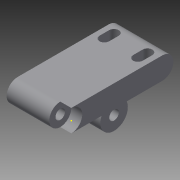
# Autodesk Inventor part: armv2
Saved by Autodesk Inventor 2015 (Build 190159000, 159)
## iProperties
Created: 2015-02-01
Part Number: armv2
Material: Generic
Document SubType Name: Modeling
Designer: Jumziey
Density: 1 g/cm^3
Appearance: Default
Author: Jumziey
Autodesk Inventor part; units mm, degrees
ref_plane "XZ Plane" through (0, 0, 0) normal (0, 1, 0) x (-1, 0, 0)
ref_plane "XY Plane" through (0, 0, 0) normal (0, 0, 1) x (1, 0, 0)
sketch "Sketch1" plane through (0, 0, 0) normal (1, 0, 0) x (0, 1, 0)
  circle A0 centre (0, 0) radius 1.75
  arc A1 (0, 4) -> (0, -4) centre (0, 0) ccw
  line L0 (0, 0) -> (15.55, 0) construction
  line L1 (15.55, -4) -> (15.55, -6) construction
  line L2 (15.55, 0) -> (33.1, 0) construction
  arc A2 (33.1, -4) -> (33.1, 4) centre (33.1, 0) ccw
  line L3 (0, 4) -> (33.1, 4)
  arc A3 (10.9674, -4) -> (20.1326, -4) centre (15.55, -6) ccw
  circle A4 centre (15.55, -6) radius 1.75
  line L4 (0, -4) -> (10.9674, -4)
  line L5 (20.1326, -4) -> (33.1, -4)
  dimension "d0" = 3.5
  dimension "d1" = 8
  dimension "d2" = 15.55
  dimension "d4" = 17.55
  dimension "d5" = 8
  dimension "d6" = 10
  dimension "d7" = 10
  dimension "d9" = 3.5
  dimension "d37" = 15.55
  constraints: 12 end point, 6 point on circle, 5 centre point, 5 coincident, 5 tangent, 3 horizontal
  measures "d0" diameter of A0
  measures "d1" diameter of A1
  measures "d2" distance of L0.start L0.end
  measures "d4" distance of L0.end L2.end
  measures "d5" diameter of A2
  measures "d6" diameter of A3
  measures "d7" distance from line of L1.end L3
  measures "d9" diameter of A4
  measures "d37" horizontal distance of point (0, 0) L1.end
extrude "Extrusion1" add sketch "Sketch1" along normal blind 6.8
sketch "Sketch2" plane through (6.8, 0, 0) normal (1, 0, 0) x (0, 0, -1)
  line L0 (0, 15.55) -> (6, 15.55) construction
  arc A0 (4, 22.7784) -> (4, 8.3216) centre (6, 15.55) ccw
  arc A1 (-4, 0) -> (4, 0) centre (0, 0) ccw construction
  line L1 (4, 0) -> (4, 8.3216) construction
  arc A2 (4, 33.1) -> (-4, 33.1) centre (0, 33.1) ccw construction
  line L2 (4, 22.7784) -> (4, 33.1) construction
  circle A3 centre (0, 0) radius 1.75
  arc A4 (-4, 0) -> (4, 0) centre (0, 0) ccw
  arc A5 (4, 33.1) -> (-4, 33.1) centre (0, 33.1) ccw
  line L3 (-4, 33.1) -> (-4, 0)
  line L4 (4, 0) -> (4, 8.3216)
  line L5 (-4, 33.1) -> (-4, 0) projected
  line L6 (4, 22.7784) -> (4, 33.1)
  dimension "d12" = 15.55
  dimension "d14" = 15
  dimension "d39" = 10
  constraints: 16 end point, 6 point on circle, 4 centre point, 4 coincident, 3 tangent, 1 parallel, 1 point on line, 1 vertical
  measures "d12" distance of point (0, 0) L0.start
  measures "d14" diameter of A0
  measures "d39" distance from line of L3 L0.end
extrude "Extrusion2" add sketch "Sketch2" along normal blind 6.4
ref_plane "Work Plane1" through (12.7, 0, 0) normal (1, 0, 0) x (0, 1, 0)
sketch "Sketch3" plane through (12.7, 0, 0) normal (1, 0, 0) x (0, 1, 0)
  circle A0 centre (0, 0) radius 1.75
  arc A1 (0, 4) -> (0, -4) centre (0, 0) ccw
  line L0 (0, 0) -> (15.55, 0) construction
  line L1 (15.55, -4) -> (15.55, -6) construction
  line L2 (15.55, 0) -> (33.1, 0) construction
  arc A2 (33.1, -4) -> (33.1, 4) centre (33.1, 0) ccw
  line L3 (0, 4) -> (33.1, 4)
  arc A3 (10.9674, -4) -> (20.1326, -4) centre (15.55, -6) ccw
  circle A4 centre (15.55, -6) radius 1.75
  line L4 (0, -4) -> (10.9674, -4)
  line L5 (20.1326, -4) -> (33.1, -4)
  dimension "d18" = 3.5
  dimension "d19" = 8
  dimension "d20" = 15.55
  dimension "d21" = 17.55
  dimension "d22" = 8
  dimension "d23" = 10
  dimension "d24" = 10
  dimension "d26" = 3.5
  dimension "d38" = 15.55
  constraints: 12 end point, 6 point on circle, 5 centre point, 5 coincident, 5 tangent, 3 horizontal
  measures "d18" diameter of A0
  measures "d19" diameter of A1
  measures "d20" distance of L0.start L0.end
  measures "d21" distance of L0.end L2.end
  measures "d22" diameter of A2
  measures "d23" diameter of A3
  measures "d24" distance from line of L1.end L3
  measures "d26" diameter of A4
  measures "d38" horizontal distance of point (0, 0) L1.end
extrude "Extrusion3" add sketch "Sketch3" along normal blind 6.8
sketch "Sketch4" plane through (0, 0, 4) normal (0, 0, 1) x (1, 0, 0)
  arc A0 (5.4, 31.35) -> (1.9, 31.35) centre (3.65, 31.35) ccw
  arc A1 (17.6, 31.35) -> (14.1, 31.35) centre (15.85, 31.35) ccw
  line L0 (0, 33.1) -> (0, 0) projected
  line L1 (0, 33.1) -> (19.5, 33.1) projected
  line L2 (19.5, 33.1) -> (19.5, 0) projected
  arc A2 (14.1, 27.85) -> (17.6, 27.85) centre (15.85, 27.85) ccw
  arc A3 (1.9, 27.85) -> (5.4, 27.85) centre (3.65, 27.85) ccw
  line L3 (17.6, 31.35) -> (17.6, 27.85)
  line L4 (14.1, 31.35) -> (14.1, 27.85)
  line L5 (5.4, 31.35) -> (5.4, 27.85)
  line L6 (1.9, 27.85) -> (1.9, 31.35)
  line L7 (0, 20.1326) -> (0, 33.1) projected
  dimension "d29" = 3.5
  dimension "d30" = 3.5
  dimension "d31" = 3.65
  dimension "d32" = 3.65
  dimension "d47" = 3.5
  dimension "d48" = 3.5
  dimension "d49" = 3.65
  dimension "d50" = 3.65
  constraints: 9 tangent, 8 end point, 8 point on circle, 4 centre point, 2 vertical, 1 parallel
  measures "d29" diameter of A0
  measures "d30" diameter of A1
  measures "d31" distance from line of A0.centre L0
  measures "d32" distance from line of L2 A1.centre
  measures "d47" diameter of A2
  measures "d48" diameter of A3
  measures "d49" distance from line of L2 A2.centre
  measures "d50" distance from line of L0 A3.centre
extrude "Extrusion5" cut sketch "Sketch4" against normal blind 8
sketch "Sketch5" plane through (0, 0, 0) normal (-1, 0, 0) x (0, 0, 1)
  arc A0 (4, 33.1) -> (-4, 33.1) centre (0, 33.1) ccw projected
  line L0 (0, 37.1) -> (0, 27.1)
  line L1 (0, 27.1) -> (-4, 27.1)
  line L2 (-4, 20.1326) -> (-4, 33.1) projected
  point P0 (0, 0)
  dimension "d40" = 10
  dimension "d41" = 4
  constraints: 4 end point, 1 perpendicular, 1 point on circle, 1 point on line, 1 vertical
  measures "d40" distance of L0.start L0.end
  measures "d41" distance between parallel lines of L0 L2
extrude "Extrusion6" cut sketch "Sketch5" against normal blind 2.15
sketch "Sketch6" plane through (19.5, 0, 0) normal (1, 0, 0) x (0, 0, -1)
  point P0 (0, 0)
sketch "Sketch7" plane through (19.5, 0, 0) normal (1, 0, 0) x (0, 0, -1)
  circle A0 centre (0, 0) radius 4
  dimension "d44" = 8
  constraints: 1 centre point, 1 coincident
  measures "d44" diameter of A0
extrude "Extrusion7" cut sketch "Sketch7" against normal blind 4
sketch "Sketch8" plane through (0, 0, 0) normal (-1, 0, 0) x (0, 0, 1)
  arc A0 (-4, 20.1326) -> (-4, 10.9674) centre (-6, 15.55) ccw projected
  circle A1 centre (-6, 15.55) radius 4
  point P0 (0, 0)
  dimension "d51" = 8
  constraints: 1 centre point, 1 coincident
  measures "d51" diameter of A1
extrude "Extrusion8" cut sketch "Sketch8" against normal blind 4
body "Solid1"
